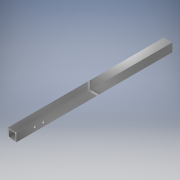
# Autodesk Inventor part: 15102898-16-P-0211
Saved by Autodesk Inventor 2017 (Build 210142000, 142)
## iProperties
Created: 2016-10-05
Part Number: 15102898-16-P-0211
Material: Aluminum 6061
Document SubType Name: Modeling
Designer: gus
Density: 2.7 g/cm^3
Appearance: Aluminum - Flat
Mass: 356.657 g
Surface Area: 837.74 cm^2
Volume: 132.095 cm^3
Author: gus
Autodesk Inventor part; units mm, degrees
ref_plane "YZ Plane" through (0, 0, 0) normal (1, 0, 0) x (0, 1, 0)
ref_plane "XZ Plane" through (0, 0, 0) normal (0, 1, 0) x (-1, 0, 0)
ref_plane "XY Plane" through (0, 0, 0) normal (0, 0, 1) x (1, 0, 0)
sketch "Sketch1" plane through (0, 0, 0) normal (0, 0, 1) x (1, 0, 0)
  line L0 (0, 0) -> (25.4, 0)
  line L1 (25.4, 0) -> (25.4, 25.4)
  line L2 (25.4, 25.4) -> (0, 25.4)
  line L3 (0, 25.4) -> (0, 0)
  line L4 (22.225, 22.225) -> (22.225, 3.175)
  line L5 (22.225, 3.175) -> (3.175, 3.175)
  line L6 (3.175, 3.175) -> (3.175, 22.225)
  line L7 (3.175, 22.225) -> (22.225, 22.225)
  dimension "d0" = 25.4
  dimension "d1" = 25.4
  dimension "d2" = 3.175
  constraints: 16 end point, 4 parallel, 2 perpendicular, 1 horizontal, 3 other
  measures "d0" distance of L2.end L1.end
  measures "d1" distance of L1.end L0.end
  measures "d2" distance between parallel lines of L1 L4
extrude "Extrusion1" add sketch "Sketch1" along normal blind 467.995
sketch "Sketch2" plane through (25.4, 0, 0) normal (1, 0, 0) x (0, 0, -1)
  line L0 (-467.995, 0) -> (-467.995, 25.4) projected
  line L1 (0, 0) -> (-467.995, 0) projected
  point P0 (-413.131, 12.7)
  point P1 (-387.731, 12.7)
  dimension "d5" = 80.264
  dimension "d6" = 25.4
  dimension "d7" = 12.7
  dimension "d8" = 12.7
  measures "d5" distance from line of L0 point (-387.731, 12.7)
  measures "d6" distance of point (-387.731, 12.7) point (-413.131, 12.7)
  measures "d7" distance from line of L1 point (-413.131, 12.7)
  measures "d8" distance from line of L1 point (-387.731, 12.7)
hole "Hole1" at (25.4, 12.7, 413.131) at (25.4, 12.7, 387.731) direction (-1, 0, 0) diameter 6.7469 end through all
body "Solid1"
